Autodesk Fusion 360 part; units mm, degrees
(part 2 of 3)
sketch "slot_guide profile (3)" plane through (0, 0, -263) normal (0, 0, 1) x (1, 0, 0) in component "cassette_2 | Top cassette | DEPTH PROVISIONAL"
  line L0 (173, 552) -> (175, 552)
  line L1 (175, 552) -> (175, 554)
  line L2 (175, 554) -> (173, 554)
  line L3 (173, 554) -> (173, 552)
  line L4 (201, 552) -> (203, 552)
  line L5 (203, 552) -> (203, 554)
  line L6 (203, 554) -> (201, 554)
  line L7 (201, 554) -> (201, 552)
  line L8 (173, 541.5) -> (175, 541.5)
  line L9 (175, 541.5) -> (175, 543.5)
  line L10 (175, 543.5) -> (173, 543.5)
  line L11 (173, 543.5) -> (173, 541.5)
  line L12 (201, 541.5) -> (203, 541.5)
  line L13 (203, 541.5) -> (203, 543.5)
  line L14 (203, 543.5) -> (201, 543.5)
  line L15 (201, 543.5) -> (201, 541.5)
  line L16 (173, 531) -> (175, 531)
  line L17 (175, 531) -> (175, 533)
  line L18 (175, 533) -> (173, 533)
  line L19 (173, 533) -> (173, 531)
  line L20 (201, 531) -> (203, 531)
  line L21 (203, 531) -> (203, 533)
  line L22 (203, 533) -> (201, 533)
  line L23 (201, 533) -> (201, 531)
  line L24 (173, 520.5) -> (175, 520.5)
  line L25 (175, 520.5) -> (175, 522.5)
  line L26 (175, 522.5) -> (173, 522.5)
  line L27 (173, 522.5) -> (173, 520.5)
  line L28 (201, 520.5) -> (203, 520.5)
  line L29 (203, 520.5) -> (203, 522.5)
  line L30 (203, 522.5) -> (201, 522.5)
  line L31 (201, 522.5) -> (201, 520.5)
  line L32 (173, 510) -> (175, 510)
  line L33 (175, 510) -> (175, 512)
  line L34 (175, 512) -> (173, 512)
  line L35 (173, 512) -> (173, 510)
  line L36 (201, 510) -> (203, 510)
  line L37 (203, 510) -> (203, 512)
  line L38 (203, 512) -> (201, 512)
  line L39 (201, 512) -> (201, 510)
  line L40 (173, 499.5) -> (175, 499.5)
  line L41 (175, 499.5) -> (175, 501.5)
  line L42 (175, 501.5) -> (173, 501.5)
  line L43 (173, 501.5) -> (173, 499.5)
  line L44 (201, 499.5) -> (203, 499.5)
  line L45 (203, 499.5) -> (203, 501.5)
  line L46 (203, 501.5) -> (201, 501.5)
  line L47 (201, 501.5) -> (201, 499.5)
  line L48 (173, 489) -> (175, 489)
  line L49 (175, 489) -> (175, 491)
  line L50 (175, 491) -> (173, 491)
  line L51 (173, 491) -> (173, 489)
  line L52 (201, 489) -> (203, 489)
  line L53 (203, 489) -> (203, 491)
  line L54 (203, 491) -> (201, 491)
  line L55 (201, 491) -> (201, 489)
  line L56 (173, 478.5) -> (175, 478.5)
  line L57 (175, 478.5) -> (175, 480.5)
  line L58 (175, 480.5) -> (173, 480.5)
  line L59 (173, 480.5) -> (173, 478.5)
  line L60 (201, 478.5) -> (203, 478.5)
  line L61 (203, 478.5) -> (203, 480.5)
  line L62 (203, 480.5) -> (201, 480.5)
  line L63 (201, 480.5) -> (201, 478.5)
  line L64 (173, 468) -> (175, 468)
  line L65 (175, 468) -> (175, 470)
  line L66 (175, 470) -> (173, 470)
  line L67 (173, 470) -> (173, 468)
  line L68 (201, 468) -> (203, 468)
  line L69 (203, 468) -> (203, 470)
  line L70 (203, 470) -> (201, 470)
  line L71 (201, 470) -> (201, 468)
  line L72 (173, 457.5) -> (175, 457.5)
  line L73 (175, 457.5) -> (175, 459.5)
  line L74 (175, 459.5) -> (173, 459.5)
  line L75 (173, 459.5) -> (173, 457.5)
  line L76 (201, 457.5) -> (203, 457.5)
  line L77 (203, 457.5) -> (203, 459.5)
  line L78 (203, 459.5) -> (201, 459.5)
  line L79 (201, 459.5) -> (201, 457.5)
  line L80 (207, 552) -> (209, 552)
  line L81 (209, 552) -> (209, 554)
  line L82 (209, 554) -> (207, 554)
  line L83 (207, 554) -> (207, 552)
  line L84 (235, 552) -> (237, 552)
  line L85 (237, 552) -> (237, 554)
  line L86 (237, 554) -> (235, 554)
  line L87 (235, 554) -> (235, 552)
  line L88 (207, 541.5) -> (209, 541.5)
  line L89 (209, 541.5) -> (209, 543.5)
  line L90 (209, 543.5) -> (207, 543.5)
  line L91 (207, 543.5) -> (207, 541.5)
  line L92 (235, 541.5) -> (237, 541.5)
  line L93 (237, 541.5) -> (237, 543.5)
  line L94 (237, 543.5) -> (235, 543.5)
  line L95 (235, 543.5) -> (235, 541.5)
  line L96 (207, 531) -> (209, 531)
  line L97 (209, 531) -> (209, 533)
  line L98 (209, 533) -> (207, 533)
  line L99 (207, 533) -> (207, 531)
  line L100 (235, 531) -> (237, 531)
  line L101 (237, 531) -> (237, 533)
  line L102 (237, 533) -> (235, 533)
  line L103 (235, 533) -> (235, 531)
  line L104 (207, 520.5) -> (209, 520.5)
  line L105 (209, 520.5) -> (209, 522.5)
  line L106 (209, 522.5) -> (207, 522.5)
  line L107 (207, 522.5) -> (207, 520.5)
  line L108 (235, 520.5) -> (237, 520.5)
  line L109 (237, 520.5) -> (237, 522.5)
  line L110 (237, 522.5) -> (235, 522.5)
  line L111 (235, 522.5) -> (235, 520.5)
  line L112 (207, 510) -> (209, 510)
  line L113 (209, 510) -> (209, 512)
  line L114 (209, 512) -> (207, 512)
  line L115 (207, 512) -> (207, 510)
  line L116 (235, 510) -> (237, 510)
  line L117 (237, 510) -> (237, 512)
  line L118 (237, 512) -> (235, 512)
  line L119 (235, 512) -> (235, 510)
  line L120 (207, 499.5) -> (209, 499.5)
  line L121 (209, 499.5) -> (209, 501.5)
  line L122 (209, 501.5) -> (207, 501.5)
  line L123 (207, 501.5) -> (207, 499.5)
  line L124 (235, 499.5) -> (237, 499.5)
  line L125 (237, 499.5) -> (237, 501.5)
  line L126 (237, 501.5) -> (235, 501.5)
  line L127 (235, 501.5) -> (235, 499.5)
  line L128 (207, 489) -> (209, 489)
  line L129 (209, 489) -> (209, 491)
  line L130 (209, 491) -> (207, 491)
  line L131 (207, 491) -> (207, 489)
  line L132 (235, 489) -> (237, 489)
  line L133 (237, 489) -> (237, 491)
  line L134 (237, 491) -> (235, 491)
  line L135 (235, 491) -> (235, 489)
  line L136 (207, 478.5) -> (209, 478.5)
  line L137 (209, 478.5) -> (209, 480.5)
  line L138 (209, 480.5) -> (207, 480.5)
  line L139 (207, 480.5) -> (207, 478.5)
  line L140 (235, 478.5) -> (237, 478.5)
  line L141 (237, 478.5) -> (237, 480.5)
  line L142 (237, 480.5) -> (235, 480.5)
  line L143 (235, 480.5) -> (235, 478.5)
  line L144 (207, 468) -> (209, 468)
  line L145 (209, 468) -> (209, 470)
  line L146 (209, 470) -> (207, 470)
  line L147 (207, 470) -> (207, 468)
  line L148 (235, 468) -> (237, 468)
  line L149 (237, 468) -> (237, 470)
  line L150 (237, 470) -> (235, 470)
  line L151 (235, 470) -> (235, 468)
  line L152 (207, 457.5) -> (209, 457.5)
  line L153 (209, 457.5) -> (209, 459.5)
  line L154 (209, 459.5) -> (207, 459.5)
  line L155 (207, 459.5) -> (207, 457.5)
  line L156 (235, 457.5) -> (237, 457.5)
  line L157 (237, 457.5) -> (237, 459.5)
  line L158 (237, 459.5) -> (235, 459.5)
  line L159 (235, 459.5) -> (235, 457.5)
extrude "slot_guide solid extrusion''" add sketch "slot_guide profile (3)" along normal blind 83 separate body makes body 178 at (207, 458.8333, -207.6667) makes body 179 at (207, 469.3333, -207.6667) makes body 180 at (207, 479.8333, -207.6667) makes body 181 at (207, 490.3333, -207.6667) makes body 182 at (207, 500.8333, -207.6667) makes body 183 at (207, 511.3333, -207.6667) makes body 184 at (207, 521.8333, -207.6667) makes body 185 at (207, 532.3333, -207.6667) makes body 186 at (207, 542.8333, -207.6667) makes body 187 at (207, 553.3333, -207.6667) makes body 188 at (201, 458.8333, -207.6667) makes body 189 at (201, 469.3333, -207.6667) makes body 190 at (201, 479.8333, -207.6667) makes body 191 at (201, 490.3333, -207.6667) makes body 192 at (201, 500.8333, -207.6667) makes body 193 at (201, 511.3333, -207.6667) makes body 194 at (201, 521.8333, -207.6667) makes body 195 at (201, 532.3333, -207.6667) makes body 196 at (201, 542.8333, -207.6667) makes body 197 at (201, 553.3333, -207.6667) makes body 198 at (173, 542.8333, -207.6667) makes body 199 at (173, 532.3333, -207.6667) makes body 200 at (173, 521.8333, -207.6667) makes body 201 at (173, 511.3333, -207.6667) makes body 202 at (173, 500.8333, -207.6667) makes body 203 at (173, 490.3333, -207.6667) makes body 204 at (173, 479.8333, -207.6667) makes body 205 at (173, 469.3333, -207.6667) makes body 206 at (173, 458.8333, -207.6667) makes body 207 at (173, 553.3333, -207.6667) makes body 208 at (235, 553.3333, -207.6667) makes body 209 at (235, 542.8333, -207.6667) makes body 210 at (235, 532.3333, -207.6667) makes body 211 at (235, 521.8333, -207.6667) makes body 212 at (235, 511.3333, -207.6667) makes body 213 at (235, 500.8333, -207.6667) makes body 214 at (235, 490.3333, -207.6667) makes body 215 at (235, 479.8333, -207.6667) makes body 216 at (235, 469.3333, -207.6667) makes body 217 at (235, 458.8333, -207.6667) in component "cassette_2 | Top cassette | DEPTH PROVISIONAL"
ref_plane "WorkPlane1" through (0, 0, -62.5) normal (0, 0, 1) x (1, 0, 0) in component "imaging_stage | Imaging stage (schematic)"
sketch "stage_base profile" plane through (0, 0, -62.5) normal (0, 0, 1) x (1, 0, 0) in component "imaging_stage | Imaging stage (schematic)"
  line L0 (-145, 251) -> (15, 251)
  line L1 (15, 251) -> (15, 269)
  line L2 (15, 269) -> (-145, 269)
  line L3 (-145, 269) -> (-145, 251)
extrude "stage_base solid extrusion" add sketch "stage_base profile" along normal blind 125 separate body makes body 218 in component "imaging_stage | Imaging stage (schematic)"
ref_plane "WorkPlane2" through (0, 0, -47.5) normal (0, 0, 1) x (1, 0, 0) in component "imaging_stage | Imaging stage (schematic)"
sketch "stage_plate profile" plane through (0, 0, -47.5) normal (0, 0, 1) x (1, 0, 0) in component "imaging_stage | Imaging stage (schematic)"
  line L0 (-121.5, 273) -> (-8.5, 273)
  line L1 (-8.5, 273) -> (-8.5, 283)
  line L2 (-8.5, 283) -> (-121.5, 283)
  line L3 (-121.5, 283) -> (-121.5, 273)
extrude "stage_plate solid extrusion" add sketch "stage_plate profile" along normal blind 95 separate body makes body 219 in component "imaging_stage | Imaging stage (schematic)"
ref_plane "WorkPlane3" through (0, 0, -41.5) normal (0, 0, 1) x (1, 0, 0) in component "imaging_stage | Imaging stage (schematic)"
sketch "glass_seat profile" plane through (0, 0, -41.5) normal (0, 0, 1) x (1, 0, 0) in component "imaging_stage | Imaging stage (schematic)"
  line L0 (-81.5, 283) -> (-48.5, 283)
  line L1 (-48.5, 283) -> (-48.5, 287)
  line L2 (-48.5, 287) -> (-81.5, 287)
  line L3 (-81.5, 287) -> (-81.5, 283)
extrude "glass_seat solid extrusion" add sketch "glass_seat profile" along normal blind 83 separate body makes body 220 in component "imaging_stage | Imaging stage (schematic)"
ref_plane "WorkPlane1" through (0, 0, -17) normal (0, 0, 1) x (1, 0, 0) in component "optics | Objective and condenser (schematic)"
sketch "objective_20x_NA075 profile" plane through (0, 0, -17) normal (0, 0, 1) x (1, 0, 0) in component "optics | Objective and condenser (schematic)"
  line L0 (-82, 186) -> (-48, 186)
  line L1 (-48, 186) -> (-48, 234)
  line L2 (-48, 234) -> (-82, 234)
  line L3 (-82, 234) -> (-82, 186)
extrude "objective_20x_NA075 solid extrusion" add sketch "objective_20x_NA075 profile" along normal blind 34 separate body makes body 221 in component "optics | Objective and condenser (schematic)"
ref_plane "WorkPlane2" through (0, 0, -24) normal (0, 0, 1) x (1, 0, 0) in component "optics | Objective and condenser (schematic)"
sketch "interchangeable_condenser profile" plane through (0, 0, -24) normal (0, 0, 1) x (1, 0, 0) in component "optics | Objective and condenser (schematic)"
  line L0 (-89, 332) -> (-41, 332)
  line L1 (-41, 332) -> (-41, 358)
  line L2 (-41, 358) -> (-89, 358)
  line L3 (-89, 358) -> (-89, 332)
extrude "interchangeable_condenser solid extrusion" add sketch "interchangeable_condenser profile" along normal blind 48 separate body makes body 222 in component "optics | Objective and condenser (schematic)"
ref_plane "WorkPlane1" through (0, 0, 157) normal (0, 0, 1) x (1, 0, 0) in component "calibration_storage | Calibration-slide compartment"
sketch "Four calibration storage slides - estimated placement" plane through (0, 0, 157) normal (0, 0, 1) x (1, 0, 0) in component "calibration_storage | Calibration-slide compartment"
  line L0 (-251, 194.5) -> (-225, 194.5)
  line L1 (-225, 194.5) -> (-225, 195.5)
  line L2 (-225, 195.5) -> (-251, 195.5)
  line L3 (-251, 195.5) -> (-251, 194.5)
  line L4 (-251, 209.5) -> (-225, 209.5)
  line L5 (-225, 209.5) -> (-225, 210.5)
  line L6 (-225, 210.5) -> (-251, 210.5)
  line L7 (-251, 210.5) -> (-251, 209.5)
  line L8 (-251, 224.5) -> (-225, 224.5)
  line L9 (-225, 224.5) -> (-225, 225.5)
  line L10 (-225, 225.5) -> (-251, 225.5)
  line L11 (-251, 225.5) -> (-251, 224.5)
  line L12 (-251, 239.5) -> (-225, 239.5)
  line L13 (-225, 239.5) -> (-225, 240.5)
  line L14 (-225, 240.5) -> (-251, 240.5)
  line L15 (-251, 240.5) -> (-251, 239.5)
extrude "Calibration slides (schematic)" add sketch "Four calibration storage slides - estimated placement" along normal blind 76 separate body makes body 223 at (-233.6667, 225.5, 182.3333) makes body 224 at (-233.6667, 210.5, 182.3333) makes body 225 at (-233.6667, 195.5, 182.3333) makes body 226 at (-233.6667, 240.5, 182.3333) in component "calibration_storage | Calibration-slide compartment"
ref_plane "WorkPlane1" through (0, 0, -325) normal (0, 0, 1) x (1, 0, 0) in component "base | Base and nominal envelope | revision 0.3"
sketch "base_plate profile" plane through (0, 0, -325) normal (0, 0, 1) x (1, 0, 0) in component "base | Base and nominal envelope | revision 0.3"
  line L0 (-325, 14) -> (325, 14)
  line L1 (325, 14) -> (325, 42)
  line L2 (325, 42) -> (-325, 42)
  line L3 (-325, 42) -> (-325, 14)
extrude "base_plate native extrusion" add sketch "base_plate profile" along normal blind 650 separate body makes body 227 in component "base | Base and nominal envelope | revision 0.3"
ref_plane "WorkPlane2" through (0, 0, -325) normal (0, 0, 1) x (1, 0, 0) in component "base | Base and nominal envelope | revision 0.3"
sketch "lower_body_band profile" plane through (0, 0, -325) normal (0, 0, 1) x (1, 0, 0) in component "base | Base and nominal envelope | revision 0.3"
  line L0 (-325, 42) -> (325, 42)
  line L1 (325, 42) -> (325, 98)
  line L2 (325, 98) -> (-325, 98)
  line L3 (-325, 98) -> (-325, 42)
extrude "lower_body_band native extrusion" add sketch "lower_body_band profile" along normal blind 650 separate body makes body 228 in component "base | Base and nominal envelope | revision 0.3"
ref_plane "WorkPlane3" through (0, 0, -282.5) normal (0, 0, 1) x (1, 0, 0) in component "base | Base and nominal envelope | revision 0.3"
sketch "foot profile" plane through (0, 0, -282.5) normal (0, 0, 1) x (1, 0, 0) in component "base | Base and nominal envelope | revision 0.3"
  line L0 (-302.5, 0) -> (-267.5, 0)
  line L1 (-267.5, 0) -> (-267.5, 14)
  line L2 (-267.5, 14) -> (-302.5, 14)
  line L3 (-302.5, 14) -> (-302.5, 0)
  line L4 (267.5, 0) -> (302.5, 0)
  line L5 (302.5, 0) -> (302.5, 14)
  line L6 (302.5, 14) -> (267.5, 14)
  line L7 (267.5, 14) -> (267.5, 0)
extrude "foot native extrusion" add sketch "foot profile" along normal blind 35 separate body makes body 229 at (-279.1667, 14, -270.8333) makes body 230 at (290.8333, 14, -270.8333) in component "base | Base and nominal envelope | revision 0.3"
ref_plane "WorkPlane4" through (0, 0, 247.5) normal (0, 0, 1) x (1, 0, 0) in component "base | Base and nominal envelope | revision 0.3"
sketch "foot profile (1)" plane through (0, 0, 247.5) normal (0, 0, 1) x (1, 0, 0) in component "base | Base and nominal envelope | revision 0.3"
  line L0 (-302.5, 0) -> (-267.5, 0)
  line L1 (-267.5, 0) -> (-267.5, 14)
  line L2 (-267.5, 14) -> (-302.5, 14)
  line L3 (-302.5, 14) -> (-302.5, 0)
  line L4 (267.5, 0) -> (302.5, 0)
  line L5 (302.5, 0) -> (302.5, 14)
  line L6 (302.5, 14) -> (267.5, 14)
  line L7 (267.5, 14) -> (267.5, 0)
extrude "foot native extrusion (1)" add sketch "foot profile (1)" along normal blind 35 separate body makes body 231 at (-279.1667, 14, 259.1667) makes body 232 at (290.8333, 14, 259.1667) in component "base | Base and nominal envelope | revision 0.3"
ref_plane "WorkPlane1" through (0, 0, -311) normal (0, 0, 1) x (1, 0, 0) in component "enclosure | Enclosure - revised silhouette | revision 0.3"
sketch "rounded_casing measured-outline reference" plane through (0, 0, -311) normal (0, 0, 1) x (1, 0, 0) in component "enclosure | Enclosure - revised silhouette | revision 0.3"
  line L0 (-325, 70) -> (325, 70)
  line L1 (325, 70) -> (325, 610)
  arc A0 (325, 610) -> (235, 700) centre (235, 610) ccw
  line L2 (235, 700) -> (-325, 700)
  line L3 (-325, 700) -> (-325, 70)
  line L4 (-311, 84) -> (-311, 686)
  line L5 (-311, 686) -> (235, 686)
  arc A1 (311, 610) -> (235, 686) centre (235, 610) ccw
  line L6 (311, 610) -> (311, 84)
  line L7 (311, 84) -> (-311, 84)
extrude "rounded_casing native extrusion" add sketch "rounded_casing measured-outline reference" along normal blind 636 separate body makes body 233 in component "enclosure | Enclosure - revised silhouette | revision 0.3"
ref_plane "WorkPlane2" through (0, 0, -325) normal (0, 0, 1) x (1, 0, 0) in component "enclosure | Enclosure - revised silhouette | revision 0.3"
sketch "rear_panel measured-outline reference" plane through (0, 0, -325) normal (0, 0, 1) x (1, 0, 0) in component "enclosure | Enclosure - revised silhouette | revision 0.3"
  line L0 (-325, 70) -> (325, 70)
  line L1 (325, 70) -> (325, 610)
  arc A0 (325, 610) -> (235, 700) centre (235, 610) ccw
  line L2 (235, 700) -> (-325, 700)
  line L3 (-325, 700) -> (-325, 70)
extrude "rear_panel native extrusion" add sketch "rear_panel measured-outline reference" along normal blind 14 separate body makes body 234 in component "enclosure | Enclosure - revised silhouette | revision 0.3"
ref_plane "WorkPlane3" through (0, 0, 325) normal (0, 0, 1) x (1, 0, 0) in component "enclosure | Enclosure - revised silhouette | revision 0.3"
sketch "front_perimeter measured-outline reference" plane through (0, 0, 325) normal (0, 0, 1) x (1, 0, 0) in component "enclosure | Enclosure - revised silhouette | revision 0.3"
  line L0 (-325, 70) -> (325, 70)
  line L1 (325, 70) -> (325, 610)
  arc A0 (325, 610) -> (235, 700) centre (235, 610) ccw
  line L2 (235, 700) -> (-325, 700)
  line L3 (-325, 700) -> (-325, 70)
  line L4 (-311, 84) -> (-311, 686)
  line L5 (-311, 686) -> (235, 686)
  arc A1 (311, 610) -> (235, 686) centre (235, 610) ccw
  line L6 (311, 610) -> (311, 84)
  line L7 (311, 84) -> (-311, 84)
extrude "front_perimeter native extrusion" add sketch "front_perimeter measured-outline reference" along normal blind 7 separate body makes body 235 in component "enclosure | Enclosure - revised silhouette | revision 0.3"
ref_plane "WorkPlane4" through (0, 0, 346) normal (0, 0, 1) x (1, 0, 0) in component "enclosure | Enclosure - revised silhouette | revision 0.3"
sketch "fixed_front_notched measured-outline reference" plane through (0, 0, 346) normal (0, 0, 1) x (1, 0, 0) in component "enclosure | Enclosure - revised silhouette | revision 0.3"
  line L0 (-311, 119) -> (62, 119)
  line L1 (62, 119) -> (62, 333)
  line L2 (62, 333) -> (30, 365)
  line L3 (30, 365) -> (30, 475)
  line L4 (30, 475) -> (62, 507)
  line L5 (62, 507) -> (62, 686)
  line L6 (62, 686) -> (-311, 686)
  line L7 (-311, 686) -> (-311, 119)
extrude "fixed_front_notched native extrusion" add sketch "fixed_front_notched measured-outline reference" along normal blind 8 separate body makes body 236 in component "enclosure | Enclosure - revised silhouette | revision 0.3"
ref_plane "WorkPlane5" through (0, 0, 325) normal (0, 0, 1) x (1, 0, 0) in component "enclosure | Enclosure - revised silhouette | revision 0.3"
sketch "front_sill profile" plane through (0, 0, 325) normal (0, 0, 1) x (1, 0, 0) in component "enclosure | Enclosure - revised silhouette | revision 0.3"
  line L0 (-325, 98) -> (325, 98)
  line L1 (325, 98) -> (325, 119)
  line L2 (325, 119) -> (-325, 119)
  line L3 (-325, 119) -> (-325, 98)
extrude "front_sill native extrusion" add sketch "front_sill profile" along normal blind 22 separate body makes body 237 in component "enclosure | Enclosure - revised silhouette | revision 0.3"
ref_plane "WorkPlane6" through (0, 0, 308) normal (0, 0, 1) x (1, 0, 0) in component "enclosure | Enclosure - revised silhouette | revision 0.3"
sketch "left_service_hinge profile" plane through (0, 0, 308) normal (0, 0, 1) x (1, 0, 0) in component "enclosure | Enclosure - revised silhouette | revision 0.3"
  line L0 (-343, 131) -> (-321, 131)
  line L1 (-321, 131) -> (-321, 159)
  line L2 (-321, 159) -> (-343, 159)
  line L3 (-343, 159) -> (-343, 131)
  line L4 (-343, 606) -> (-321, 606)
  line L5 (-321, 606) -> (-321, 634)
  line L6 (-321, 634) -> (-343, 634)
  line L7 (-343, 634) -> (-343, 606)
extrude "left_service_hinge native extrusion" add sketch "left_service_hinge profile" along normal blind 12 separate body makes body 238 at (-335.6667, 140.3333, 308) makes body 239 at (-335.6667, 615.3333, 308) in component "enclosure | Enclosure - revised silhouette | revision 0.3"
ref_plane "WorkPlane7" through (0, 0, 227.5) normal (0, 0, 1) x (1, 0, 0) in component "enclosure | Enclosure - revised silhouette | revision 0.3"
sketch "right_service_latch profile" plane through (0, 0, 227.5) normal (0, 0, 1) x (1, 0, 0) in component "enclosure | Enclosure - revised silhouette | revision 0.3"
  line L0 (325, 137.5) -> (342, 137.5)
  line L1 (342, 137.5) -> (342, 152.5)
  line L2 (342, 152.5) -> (325, 152.5)
  line L3 (325, 152.5) -> (325, 137.5)
  line L4 (325, 612.5) -> (342, 612.5)
  line L5 (342, 612.5) -> (342, 627.5)
  line L6 (342, 627.5) -> (325, 627.5)
  line L7 (325, 627.5) -> (325, 612.5)
extrude "right_service_latch native extrusion" add sketch "right_service_latch profile" along normal blind 25 separate body makes body 240 at (336.3333, 152.5, 235.8333) makes body 241 at (336.3333, 627.5, 235.8333) in component "enclosure | Enclosure - revised silhouette | revision 0.3"
ref_plane "WorkPlane8" through (0, 0, -296) normal (0, 0, 1) x (1, 0, 0) in component "enclosure | Enclosure - revised silhouette | revision 0.3"
sketch "right_service_panel profile" plane through (0, 0, -296) normal (0, 0, 1) x (1, 0, 0) in component "enclosure | Enclosure - revised silhouette | revision 0.3"
  line L0 (324, 129) -> (326, 129)
  line L1 (326, 129) -> (326, 537)
  line L2 (326, 537) -> (324, 537)
  line L3 (324, 537) -> (324, 129)
extrude "right_service_panel native extrusion" add sketch "right_service_panel profile" along normal blind 410 separate body makes body 242 in component "enclosure | Enclosure - revised silhouette | revision 0.3"
ref_plane "WorkPlane9" through (0, 0, -19) normal (0, 0, 1) x (1, 0, 0) in component "enclosure | Enclosure - revised silhouette | revision 0.3"
sketch "right_service_handle profile" plane through (0, 0, -19) normal (0, 0, 1) x (1, 0, 0) in component "enclosure | Enclosure - revised silhouette | revision 0.3"
  line L0 (326, 305.5) -> (338, 305.5)
  line L1 (338, 305.5) -> (338, 390.5)
  line L2 (338, 390.5) -> (326, 390.5)
  line L3 (326, 390.5) -> (326, 305.5)
extrude "right_service_handle native extrusion" add sketch "right_service_handle profile" along normal blind 24 separate body makes body 243 in component "enclosure | Enclosure - revised silhouette | revision 0.3"
ref_plane "WorkPlane10" through (0, 0, -282.5) normal (0, 0, 1) x (1, 0, 0) in component "enclosure | Enclosure - revised silhouette | revision 0.3"
sketch "side_vent profile" plane through (0, 0, -282.5) normal (0, 0, 1) x (1, 0, 0) in component "enclosure | Enclosure - revised silhouette | revision 0.3"
  line L0 (324.5, 106.5) -> (326.5, 106.5)
  line L1 (326.5, 106.5) -> (326.5, 109.5)
  line L2 (326.5, 109.5) -> (324.5, 109.5)
  line L3 (324.5, 109.5) -> (324.5, 106.5)
  line L4 (324.5, 117.5) -> (326.5, 117.5)
  line L5 (326.5, 117.5) -> (326.5, 120.5)
  line L6 (326.5, 120.5) -> (324.5, 120.5)
  line L7 (324.5, 120.5) -> (324.5, 117.5)
  line L8 (324.5, 128.5) -> (326.5, 128.5)
  line L9 (326.5, 128.5) -> (326.5, 131.5)
  line L10 (326.5, 131.5) -> (324.5, 131.5)
  line L11 (324.5, 131.5) -> (324.5, 128.5)
  line L12 (324.5, 139.5) -> (326.5, 139.5)
  line L13 (326.5, 139.5) -> (326.5, 142.5)
  line L14 (326.5, 142.5) -> (324.5, 142.5)
  line L15 (324.5, 142.5) -> (324.5, 139.5)
  line L16 (324.5, 150.5) -> (326.5, 150.5)
  line L17 (326.5, 150.5) -> (326.5, 153.5)
  line L18 (326.5, 153.5) -> (324.5, 153.5)
  line L19 (324.5, 153.5) -> (324.5, 150.5)
extrude "side_vent native extrusion" add sketch "side_vent profile" along normal blind 5 separate body makes body 244 at (324.5, 141.5, -280.8333) makes body 245 at (324.5, 130.5, -280.8333) makes body 246 at (324.5, 119.5, -280.8333) makes body 247 at (324.5, 108.5, -280.8333) makes body 248 at (324.5, 152.5, -280.8333) in component "enclosure | Enclosure - revised silhouette | revision 0.3"
ref_plane "WorkPlane11" through (0, 0, -254.5) normal (0, 0, 1) x (1, 0, 0) in component "enclosure | Enclosure - revised silhouette | revision 0.3"
sketch "side_vent profile (1)" plane through (0, 0, -254.5) normal (0, 0, 1) x (1, 0, 0) in component "enclosure | Enclosure - revised silhouette | revision 0.3"
  line L0 (324.5, 106.5) -> (326.5, 106.5)
  line L1 (326.5, 106.5) -> (326.5, 109.5)
  line L2 (326.5, 109.5) -> (324.5, 109.5)
  line L3 (324.5, 109.5) -> (324.5, 106.5)
  line L4 (324.5, 117.5) -> (326.5, 117.5)
  line L5 (326.5, 117.5) -> (326.5, 120.5)
  line L6 (326.5, 120.5) -> (324.5, 120.5)
  line L7 (324.5, 120.5) -> (324.5, 117.5)
  line L8 (324.5, 128.5) -> (326.5, 128.5)
  line L9 (326.5, 128.5) -> (326.5, 131.5)
  line L10 (326.5, 131.5) -> (324.5, 131.5)
  line L11 (324.5, 131.5) -> (324.5, 128.5)
  line L12 (324.5, 139.5) -> (326.5, 139.5)
  line L13 (326.5, 139.5) -> (326.5, 142.5)
  line L14 (326.5, 142.5) -> (324.5, 142.5)
  line L15 (324.5, 142.5) -> (324.5, 139.5)
  line L16 (324.5, 150.5) -> (326.5, 150.5)
  line L17 (326.5, 150.5) -> (326.5, 153.5)
  line L18 (326.5, 153.5) -> (324.5, 153.5)
  line L19 (324.5, 153.5) -> (324.5, 150.5)
extrude "side_vent native extrusion (1)" add sketch "side_vent profile (1)" along normal blind 5 separate body makes body 249 at (324.5, 141.5, -252.8333) makes body 250 at (324.5, 130.5, -252.8333) makes body 251 at (324.5, 119.5, -252.8333) makes body 252 at (324.5, 108.5, -252.8333) makes body 253 at (324.5, 152.5, -252.8333) in component "enclosure | Enclosure - revised silhouette | revision 0.3"
ref_plane "WorkPlane12" through (0, 0, -226.5) normal (0, 0, 1) x (1, 0, 0) in component "enclosure | Enclosure - revised silhouette | revision 0.3"
sketch "side_vent profile (2)" plane through (0, 0, -226.5) normal (0, 0, 1) x (1, 0, 0) in component "enclosure | Enclosure - revised silhouette | revision 0.3"
  line L0 (324.5, 106.5) -> (326.5, 106.5)
  line L1 (326.5, 106.5) -> (326.5, 109.5)
  line L2 (326.5, 109.5) -> (324.5, 109.5)
  line L3 (324.5, 109.5) -> (324.5, 106.5)
  line L4 (324.5, 117.5) -> (326.5, 117.5)
  line L5 (326.5, 117.5) -> (326.5, 120.5)
  line L6 (326.5, 120.5) -> (324.5, 120.5)
  line L7 (324.5, 120.5) -> (324.5, 117.5)
  line L8 (324.5, 128.5) -> (326.5, 128.5)
  line L9 (326.5, 128.5) -> (326.5, 131.5)
  line L10 (326.5, 131.5) -> (324.5, 131.5)
  line L11 (324.5, 131.5) -> (324.5, 128.5)
  line L12 (324.5, 139.5) -> (326.5, 139.5)
  line L13 (326.5, 139.5) -> (326.5, 142.5)
  line L14 (326.5, 142.5) -> (324.5, 142.5)
  line L15 (324.5, 142.5) -> (324.5, 139.5)
  line L16 (324.5, 150.5) -> (326.5, 150.5)
  line L17 (326.5, 150.5) -> (326.5, 153.5)
  line L18 (326.5, 153.5) -> (324.5, 153.5)
  line L19 (324.5, 153.5) -> (324.5, 150.5)
extrude "side_vent native extrusion (2)" add sketch "side_vent profile (2)" along normal blind 5 separate body makes body 254 at (324.5, 141.5, -224.8333) makes body 255 at (324.5, 130.5, -224.8333) makes body 256 at (324.5, 119.5, -224.8333) makes body 257 at (324.5, 108.5, -224.8333) makes body 258 at (324.5, 152.5, -224.8333) in component "enclosure | Enclosure - revised silhouette | revision 0.3"
ref_plane "WorkPlane13" through (0, 0, -198.5) normal (0, 0, 1) x (1, 0, 0) in component "enclosure | Enclosure - revised silhouette | revision 0.3"
sketch "side_vent profile (3)" plane through (0, 0, -198.5) normal (0, 0, 1) x (1, 0, 0) in component "enclosure | Enclosure - revised silhouette | revision 0.3"
  line L0 (324.5, 106.5) -> (326.5, 106.5)
  line L1 (326.5, 106.5) -> (326.5, 109.5)
  line L2 (326.5, 109.5) -> (324.5, 109.5)
  line L3 (324.5, 109.5) -> (324.5, 106.5)
  line L4 (324.5, 117.5) -> (326.5, 117.5)
  line L5 (326.5, 117.5) -> (326.5, 120.5)
  line L6 (326.5, 120.5) -> (324.5, 120.5)
  line L7 (324.5, 120.5) -> (324.5, 117.5)
  line L8 (324.5, 128.5) -> (326.5, 128.5)
  line L9 (326.5, 128.5) -> (326.5, 131.5)
  line L10 (326.5, 131.5) -> (324.5, 131.5)
  line L11 (324.5, 131.5) -> (324.5, 128.5)
  line L12 (324.5, 139.5) -> (326.5, 139.5)
  line L13 (326.5, 139.5) -> (326.5, 142.5)
  line L14 (326.5, 142.5) -> (324.5, 142.5)
  line L15 (324.5, 142.5) -> (324.5, 139.5)
  line L16 (324.5, 150.5) -> (326.5, 150.5)
  line L17 (326.5, 150.5) -> (326.5, 153.5)
  line L18 (326.5, 153.5) -> (324.5, 153.5)
  line L19 (324.5, 153.5) -> (324.5, 150.5)
extrude "side_vent native extrusion (3)" add sketch "side_vent profile (3)" along normal blind 5 separate body makes body 259 at (324.5, 141.5, -196.8333) makes body 260 at (324.5, 130.5, -196.8333) makes body 261 at (324.5, 119.5, -196.8333) makes body 262 at (324.5, 108.5, -196.8333) makes body 263 at (324.5, 152.5, -196.8333) in component "enclosure | Enclosure - revised silhouette | revision 0.3"
ref_plane "WorkPlane14" through (0, 0, -170.5) normal (0, 0, 1) x (1, 0, 0) in component "enclosure | Enclosure - revised silhouette | revision 0.3"
sketch "side_vent profile (4)" plane through (0, 0, -170.5) normal (0, 0, 1) x (1, 0, 0) in component "enclosure | Enclosure - revised silhouette | revision 0.3"
  line L0 (324.5, 106.5) -> (326.5, 106.5)
  line L1 (326.5, 106.5) -> (326.5, 109.5)
  line L2 (326.5, 109.5) -> (324.5, 109.5)
  line L3 (324.5, 109.5) -> (324.5, 106.5)
  line L4 (324.5, 117.5) -> (326.5, 117.5)
  line L5 (326.5, 117.5) -> (326.5, 120.5)
  line L6 (326.5, 120.5) -> (324.5, 120.5)
  line L7 (324.5, 120.5) -> (324.5, 117.5)
  line L8 (324.5, 128.5) -> (326.5, 128.5)
  line L9 (326.5, 128.5) -> (326.5, 131.5)
  line L10 (326.5, 131.5) -> (324.5, 131.5)
  line L11 (324.5, 131.5) -> (324.5, 128.5)
  line L12 (324.5, 139.5) -> (326.5, 139.5)
  line L13 (326.5, 139.5) -> (326.5, 142.5)
  line L14 (326.5, 142.5) -> (324.5, 142.5)
  line L15 (324.5, 142.5) -> (324.5, 139.5)
  line L16 (324.5, 150.5) -> (326.5, 150.5)
  line L17 (326.5, 150.5) -> (326.5, 153.5)
  line L18 (326.5, 153.5) -> (324.5, 153.5)
  line L19 (324.5, 153.5) -> (324.5, 150.5)
extrude "side_vent native extrusion (4)" add sketch "side_vent profile (4)" along normal blind 5 separate body makes body 264 at (324.5, 141.5, -168.8333) makes body 265 at (324.5, 130.5, -168.8333) makes body 266 at (324.5, 119.5, -168.8333) makes body 267 at (324.5, 108.5, -168.8333) makes body 268 at (324.5, 152.5, -168.8333) in component "enclosure | Enclosure - revised silhouette | revision 0.3"
ref_plane "WorkPlane15" through (0, 0, -142.5) normal (0, 0, 1) x (1, 0, 0) in component "enclosure | Enclosure - revised silhouette | revision 0.3"
sketch "side_vent profile (5)" plane through (0, 0, -142.5) normal (0, 0, 1) x (1, 0, 0) in component "enclosure | Enclosure - revised silhouette | revision 0.3"
  line L0 (324.5, 106.5) -> (326.5, 106.5)
  line L1 (326.5, 106.5) -> (326.5, 109.5)
  line L2 (326.5, 109.5) -> (324.5, 109.5)
  line L3 (324.5, 109.5) -> (324.5, 106.5)
  line L4 (324.5, 117.5) -> (326.5, 117.5)
  line L5 (326.5, 117.5) -> (326.5, 120.5)
  line L6 (326.5, 120.5) -> (324.5, 120.5)
  line L7 (324.5, 120.5) -> (324.5, 117.5)
  line L8 (324.5, 128.5) -> (326.5, 128.5)
  line L9 (326.5, 128.5) -> (326.5, 131.5)
  line L10 (326.5, 131.5) -> (324.5, 131.5)
  line L11 (324.5, 131.5) -> (324.5, 128.5)
  line L12 (324.5, 139.5) -> (326.5, 139.5)
  line L13 (326.5, 139.5) -> (326.5, 142.5)
  line L14 (326.5, 142.5) -> (324.5, 142.5)
  line L15 (324.5, 142.5) -> (324.5, 139.5)
  line L16 (324.5, 150.5) -> (326.5, 150.5)
  line L17 (326.5, 150.5) -> (326.5, 153.5)
  line L18 (326.5, 153.5) -> (324.5, 153.5)
  line L19 (324.5, 153.5) -> (324.5, 150.5)
extrude "side_vent native extrusion (5)" add sketch "side_vent profile (5)" along normal blind 5 separate body makes body 269 at (324.5, 141.5, -140.8333) makes body 270 at (324.5, 130.5, -140.8333) makes body 271 at (324.5, 119.5, -140.8333) makes body 272 at (324.5, 108.5, -140.8333) makes body 273 at (324.5, 152.5, -140.8333) in component "enclosure | Enclosure - revised silhouette | revision 0.3"
ref_plane "WorkPlane16" through (0, 0, -114.5) normal (0, 0, 1) x (1, 0, 0) in component "enclosure | Enclosure - revised silhouette | revision 0.3"
sketch "side_vent profile (6)" plane through (0, 0, -114.5) normal (0, 0, 1) x (1, 0, 0) in component "enclosure | Enclosure - revised silhouette | revision 0.3"
  line L0 (324.5, 106.5) -> (326.5, 106.5)
  line L1 (326.5, 106.5) -> (326.5, 109.5)
  line L2 (326.5, 109.5) -> (324.5, 109.5)
  line L3 (324.5, 109.5) -> (324.5, 106.5)
  line L4 (324.5, 117.5) -> (326.5, 117.5)
  line L5 (326.5, 117.5) -> (326.5, 120.5)
  line L6 (326.5, 120.5) -> (324.5, 120.5)
  line L7 (324.5, 120.5) -> (324.5, 117.5)
  line L8 (324.5, 128.5) -> (326.5, 128.5)
  line L9 (326.5, 128.5) -> (326.5, 131.5)
  line L10 (326.5, 131.5) -> (324.5, 131.5)
  line L11 (324.5, 131.5) -> (324.5, 128.5)
  line L12 (324.5, 139.5) -> (326.5, 139.5)
  line L13 (326.5, 139.5) -> (326.5, 142.5)
  line L14 (326.5, 142.5) -> (324.5, 142.5)
  line L15 (324.5, 142.5) -> (324.5, 139.5)
  line L16 (324.5, 150.5) -> (326.5, 150.5)
  line L17 (326.5, 150.5) -> (326.5, 153.5)
  line L18 (326.5, 153.5) -> (324.5, 153.5)
  line L19 (324.5, 153.5) -> (324.5, 150.5)
extrude "side_vent native extrusion (6)" add sketch "side_vent profile (6)" along normal blind 5 separate body makes body 274 at (324.5, 141.5, -112.8333) makes body 275 at (324.5, 130.5, -112.8333) makes body 276 at (324.5, 119.5, -112.8333) makes body 277 at (324.5, 108.5, -112.8333) makes body 278 at (324.5, 152.5, -112.8333) in component "enclosure | Enclosure - revised silhouette | revision 0.3"
ref_plane "WorkPlane17" through (0, 0, -86.5) normal (0, 0, 1) x (1, 0, 0) in component "enclosure | Enclosure - revised silhouette | revision 0.3"
sketch "side_vent profile (7)" plane through (0, 0, -86.5) normal (0, 0, 1) x (1, 0, 0) in component "enclosure | Enclosure - revised silhouette | revision 0.3"
  line L0 (324.5, 106.5) -> (326.5, 106.5)
  line L1 (326.5, 106.5) -> (326.5, 109.5)
  line L2 (326.5, 109.5) -> (324.5, 109.5)
  line L3 (324.5, 109.5) -> (324.5, 106.5)
  line L4 (324.5, 117.5) -> (326.5, 117.5)
  line L5 (326.5, 117.5) -> (326.5, 120.5)
  line L6 (326.5, 120.5) -> (324.5, 120.5)
  line L7 (324.5, 120.5) -> (324.5, 117.5)
  line L8 (324.5, 128.5) -> (326.5, 128.5)
  line L9 (326.5, 128.5) -> (326.5, 131.5)
  line L10 (326.5, 131.5) -> (324.5, 131.5)
  line L11 (324.5, 131.5) -> (324.5, 128.5)
  line L12 (324.5, 139.5) -> (326.5, 139.5)
  line L13 (326.5, 139.5) -> (326.5, 142.5)
  line L14 (326.5, 142.5) -> (324.5, 142.5)
  line L15 (324.5, 142.5) -> (324.5, 139.5)
  line L16 (324.5, 150.5) -> (326.5, 150.5)
  line L17 (326.5, 150.5) -> (326.5, 153.5)
  line L18 (326.5, 153.5) -> (324.5, 153.5)
  line L19 (324.5, 153.5) -> (324.5, 150.5)
extrude "side_vent native extrusion (7)" add sketch "side_vent profile (7)" along normal blind 5 separate body makes body 279 at (324.5, 141.5, -84.8333) makes body 280 at (324.5, 130.5, -84.8333) makes body 281 at (324.5, 119.5, -84.8333) makes body 282 at (324.5, 108.5, -84.8333) makes body 283 at (324.5, 152.5, -84.8333) in component "enclosure | Enclosure - revised silhouette | revision 0.3"
ref_plane "WorkPlane18" through (0, 0, -58.5) normal (0, 0, 1) x (1, 0, 0) in component "enclosure | Enclosure - revised silhouette | revision 0.3"
sketch "side_vent profile (8)" plane through (0, 0, -58.5) normal (0, 0, 1) x (1, 0, 0) in component "enclosure | Enclosure - revised silhouette | revision 0.3"
  line L0 (324.5, 106.5) -> (326.5, 106.5)
  line L1 (326.5, 106.5) -> (326.5, 109.5)
  line L2 (326.5, 109.5) -> (324.5, 109.5)
  line L3 (324.5, 109.5) -> (324.5, 106.5)
  line L4 (324.5, 117.5) -> (326.5, 117.5)
  line L5 (326.5, 117.5) -> (326.5, 120.5)
  line L6 (326.5, 120.5) -> (324.5, 120.5)
  line L7 (324.5, 120.5) -> (324.5, 117.5)
  line L8 (324.5, 128.5) -> (326.5, 128.5)
  line L9 (326.5, 128.5) -> (326.5, 131.5)
  line L10 (326.5, 131.5) -> (324.5, 131.5)
  line L11 (324.5, 131.5) -> (324.5, 128.5)
  line L12 (324.5, 139.5) -> (326.5, 139.5)
  line L13 (326.5, 139.5) -> (326.5, 142.5)
  line L14 (326.5, 142.5) -> (324.5, 142.5)
  line L15 (324.5, 142.5) -> (324.5, 139.5)
  line L16 (324.5, 150.5) -> (326.5, 150.5)
  line L17 (326.5, 150.5) -> (326.5, 153.5)
  line L18 (326.5, 153.5) -> (324.5, 153.5)
  line L19 (324.5, 153.5) -> (324.5, 150.5)
extrude "side_vent native extrusion (8)" add sketch "side_vent profile (8)" along normal blind 5 separate body makes body 284 at (324.5, 141.5, -56.8333) makes body 285 at (324.5, 130.5, -56.8333) makes body 286 at (324.5, 119.5, -56.8333) makes body 287 at (324.5, 108.5, -56.8333) makes body 288 at (324.5, 152.5, -56.8333) in component "enclosure | Enclosure - revised silhouette | revision 0.3"
ref_plane "WorkPlane19" through (0, 0, -30.5) normal (0, 0, 1) x (1, 0, 0) in component "enclosure | Enclosure - revised silhouette | revision 0.3"
sketch "side_vent profile (9)" plane through (0, 0, -30.5) normal (0, 0, 1) x (1, 0, 0) in component "enclosure | Enclosure - revised silhouette | revision 0.3"
  line L0 (324.5, 106.5) -> (326.5, 106.5)
  line L1 (326.5, 106.5) -> (326.5, 109.5)
  line L2 (326.5, 109.5) -> (324.5, 109.5)
  line L3 (324.5, 109.5) -> (324.5, 106.5)
  line L4 (324.5, 117.5) -> (326.5, 117.5)
  line L5 (326.5, 117.5) -> (326.5, 120.5)
  line L6 (326.5, 120.5) -> (324.5, 120.5)
  line L7 (324.5, 120.5) -> (324.5, 117.5)
  line L8 (324.5, 128.5) -> (326.5, 128.5)
  line L9 (326.5, 128.5) -> (326.5, 131.5)
  line L10 (326.5, 131.5) -> (324.5, 131.5)
  line L11 (324.5, 131.5) -> (324.5, 128.5)
  line L12 (324.5, 139.5) -> (326.5, 139.5)
  line L13 (326.5, 139.5) -> (326.5, 142.5)
  line L14 (326.5, 142.5) -> (324.5, 142.5)
  line L15 (324.5, 142.5) -> (324.5, 139.5)
  line L16 (324.5, 150.5) -> (326.5, 150.5)
  line L17 (326.5, 150.5) -> (326.5, 153.5)
  line L18 (326.5, 153.5) -> (324.5, 153.5)
  line L19 (324.5, 153.5) -> (324.5, 150.5)
extrude "side_vent native extrusion (9)" add sketch "side_vent profile (9)" along normal blind 5 separate body makes body 289 at (324.5, 141.5, -28.8333) makes body 290 at (324.5, 130.5, -28.8333) makes body 291 at (324.5, 119.5, -28.8333) makes body 292 at (324.5, 108.5, -28.8333) makes body 293 at (324.5, 152.5, -28.8333) in component "enclosure | Enclosure - revised silhouette | revision 0.3"
ref_plane "WorkPlane20" through (0, 0, -2.5) normal (0, 0, 1) x (1, 0, 0) in component "enclosure | Enclosure - revised silhouette | revision 0.3"
sketch "side_vent profile (10)" plane through (0, 0, -2.5) normal (0, 0, 1) x (1, 0, 0) in component "enclosure | Enclosure - revised silhouette | revision 0.3"
  line L0 (324.5, 106.5) -> (326.5, 106.5)
  line L1 (326.5, 106.5) -> (326.5, 109.5)
  line L2 (326.5, 109.5) -> (324.5, 109.5)
  line L3 (324.5, 109.5) -> (324.5, 106.5)
  line L4 (324.5, 117.5) -> (326.5, 117.5)
  line L5 (326.5, 117.5) -> (326.5, 120.5)
  line L6 (326.5, 120.5) -> (324.5, 120.5)
  line L7 (324.5, 120.5) -> (324.5, 117.5)
  line L8 (324.5, 128.5) -> (326.5, 128.5)
  line L9 (326.5, 128.5) -> (326.5, 131.5)
  line L10 (326.5, 131.5) -> (324.5, 131.5)
  line L11 (324.5, 131.5) -> (324.5, 128.5)
  line L12 (324.5, 139.5) -> (326.5, 139.5)
  line L13 (326.5, 139.5) -> (326.5, 142.5)
  line L14 (326.5, 142.5) -> (324.5, 142.5)
  line L15 (324.5, 142.5) -> (324.5, 139.5)
  line L16 (324.5, 150.5) -> (326.5, 150.5)
  line L17 (326.5, 150.5) -> (326.5, 153.5)
  line L18 (326.5, 153.5) -> (324.5, 153.5)
  line L19 (324.5, 153.5) -> (324.5, 150.5)
extrude "side_vent native extrusion (10)" add sketch "side_vent profile (10)" along normal blind 5 separate body makes body 294 at (324.5, 141.5, -0.8333) makes body 295 at (324.5, 130.5, -0.8333) makes body 296 at (324.5, 119.5, -0.8333) makes body 297 at (324.5, 108.5, -0.8333) makes body 298 at (324.5, 152.5, -0.8333) in component "enclosure | Enclosure - revised silhouette | revision 0.3"
ref_plane "WorkPlane21" through (0, 0, 25.5) normal (0, 0, 1) x (1, 0, 0) in component "enclosure | Enclosure - revised silhouette | revision 0.3"
sketch "side_vent profile (11)" plane through (0, 0, 25.5) normal (0, 0, 1) x (1, 0, 0) in component "enclosure | Enclosure - revised silhouette | revision 0.3"
  line L0 (324.5, 106.5) -> (326.5, 106.5)
  line L1 (326.5, 106.5) -> (326.5, 109.5)
  line L2 (326.5, 109.5) -> (324.5, 109.5)
  line L3 (324.5, 109.5) -> (324.5, 106.5)
  line L4 (324.5, 117.5) -> (326.5, 117.5)
  line L5 (326.5, 117.5) -> (326.5, 120.5)
  line L6 (326.5, 120.5) -> (324.5, 120.5)
  line L7 (324.5, 120.5) -> (324.5, 117.5)
  line L8 (324.5, 128.5) -> (326.5, 128.5)
  line L9 (326.5, 128.5) -> (326.5, 131.5)
  line L10 (326.5, 131.5) -> (324.5, 131.5)
  line L11 (324.5, 131.5) -> (324.5, 128.5)
  line L12 (324.5, 139.5) -> (326.5, 139.5)
  line L13 (326.5, 139.5) -> (326.5, 142.5)
  line L14 (326.5, 142.5) -> (324.5, 142.5)
  line L15 (324.5, 142.5) -> (324.5, 139.5)
  line L16 (324.5, 150.5) -> (326.5, 150.5)
  line L17 (326.5, 150.5) -> (326.5, 153.5)
  line L18 (326.5, 153.5) -> (324.5, 153.5)
  line L19 (324.5, 153.5) -> (324.5, 150.5)
extrude "side_vent native extrusion (11)" add sketch "side_vent profile (11)" along normal blind 5 separate body makes body 299 at (324.5, 141.5, 27.1667) makes body 300 at (324.5, 130.5, 27.1667) makes body 301 at (324.5, 119.5, 27.1667) makes body 302 at (324.5, 108.5, 27.1667) makes body 303 at (324.5, 152.5, 27.1667) in component "enclosure | Enclosure - revised silhouette | revision 0.3"
ref_plane "WorkPlane22" through (0, 0, 53.5) normal (0, 0, 1) x (1, 0, 0) in component "enclosure | Enclosure - revised silhouette | revision 0.3"
sketch "side_vent profile (12)" plane through (0, 0, 53.5) normal (0, 0, 1) x (1, 0, 0) in component "enclosure | Enclosure - revised silhouette | revision 0.3"
  line L0 (324.5, 106.5) -> (326.5, 106.5)
  line L1 (326.5, 106.5) -> (326.5, 109.5)
  line L2 (326.5, 109.5) -> (324.5, 109.5)
  line L3 (324.5, 109.5) -> (324.5, 106.5)
  line L4 (324.5, 117.5) -> (326.5, 117.5)
  line L5 (326.5, 117.5) -> (326.5, 120.5)
  line L6 (326.5, 120.5) -> (324.5, 120.5)
  line L7 (324.5, 120.5) -> (324.5, 117.5)
  line L8 (324.5, 128.5) -> (326.5, 128.5)
  line L9 (326.5, 128.5) -> (326.5, 131.5)
  line L10 (326.5, 131.5) -> (324.5, 131.5)
  line L11 (324.5, 131.5) -> (324.5, 128.5)
  line L12 (324.5, 139.5) -> (326.5, 139.5)
  line L13 (326.5, 139.5) -> (326.5, 142.5)
  line L14 (326.5, 142.5) -> (324.5, 142.5)
  line L15 (324.5, 142.5) -> (324.5, 139.5)
  line L16 (324.5, 150.5) -> (326.5, 150.5)
  line L17 (326.5, 150.5) -> (326.5, 153.5)
  line L18 (326.5, 153.5) -> (324.5, 153.5)
  line L19 (324.5, 153.5) -> (324.5, 150.5)
extrude "side_vent native extrusion (12)" add sketch "side_vent profile (12)" along normal blind 5 separate body makes body 304 at (324.5, 141.5, 55.1667) makes body 305 at (324.5, 130.5, 55.1667) makes body 306 at (324.5, 119.5, 55.1667) makes body 307 at (324.5, 108.5, 55.1667) makes body 308 at (324.5, 152.5, 55.1667) in component "enclosure | Enclosure - revised silhouette | revision 0.3"
ref_plane "WorkPlane23" through (0, 0, 81.5) normal (0, 0, 1) x (1, 0, 0) in component "enclosure | Enclosure - revised silhouette | revision 0.3"
sketch "side_vent profile (13)" plane through (0, 0, 81.5) normal (0, 0, 1) x (1, 0, 0) in component "enclosure | Enclosure - revised silhouette | revision 0.3"
  line L0 (324.5, 106.5) -> (326.5, 106.5)
  line L1 (326.5, 106.5) -> (326.5, 109.5)
  line L2 (326.5, 109.5) -> (324.5, 109.5)
  line L3 (324.5, 109.5) -> (324.5, 106.5)
  line L4 (324.5, 117.5) -> (326.5, 117.5)
  line L5 (326.5, 117.5) -> (326.5, 120.5)
  line L6 (326.5, 120.5) -> (324.5, 120.5)
  line L7 (324.5, 120.5) -> (324.5, 117.5)
  line L8 (324.5, 128.5) -> (326.5, 128.5)
  line L9 (326.5, 128.5) -> (326.5, 131.5)
  line L10 (326.5, 131.5) -> (324.5, 131.5)
  line L11 (324.5, 131.5) -> (324.5, 128.5)
  line L12 (324.5, 139.5) -> (326.5, 139.5)
  line L13 (326.5, 139.5) -> (326.5, 142.5)
  line L14 (326.5, 142.5) -> (324.5, 142.5)
  line L15 (324.5, 142.5) -> (324.5, 139.5)
  line L16 (324.5, 150.5) -> (326.5, 150.5)
  line L17 (326.5, 150.5) -> (326.5, 153.5)
  line L18 (326.5, 153.5) -> (324.5, 153.5)
  line L19 (324.5, 153.5) -> (324.5, 150.5)
extrude "side_vent native extrusion (13)" add sketch "side_vent profile (13)" along normal blind 5 separate body makes body 309 at (324.5, 141.5, 83.1667) makes body 310 at (324.5, 130.5, 83.1667) makes body 311 at (324.5, 119.5, 83.1667) makes body 312 at (324.5, 108.5, 83.1667) makes body 313 at (324.5, 152.5, 83.1667) in component "enclosure | Enclosure - revised silhouette | revision 0.3"
ref_plane "WorkPlane1" through (0, 0, 347) normal (0, 0, 1) x (1, 0, 0) in component "front_controls | Front control strip | revision 0.3"
sketch "control_recess profile" plane through (0, 0, 347) normal (0, 0, 1) x (1, 0, 0) in component "front_controls | Front control strip | revision 0.3"
  line L0 (-219, 51) -> (-35, 51)
  line L1 (-35, 51) -> (-35, 87)
  line L2 (-35, 87) -> (-219, 87)
  line L3 (-219, 87) -> (-219, 51)
extrude "control_recess native extrusion" add sketch "control_recess profile" along normal blind 4 separate body makes body 314 in component "front_controls | Front control strip | revision 0.3"
ref_plane "WorkPlane2" through (0, 0, 351.5) normal (0, 0, 1) x (1, 0, 0) in component "front_controls | Front control strip | revision 0.3"
sketch "led_0 profile" plane through (0, 0, 351.5) normal (0, 0, 1) x (1, 0, 0) in component "front_controls | Front control strip | revision 0.3"
  line L0 (-141.5, 68.5) -> (-132.5, 68.5)
  line L1 (-132.5, 68.5) -> (-132.5, 77.5)
  line L2 (-132.5, 77.5) -> (-141.5, 77.5)
  line L3 (-141.5, 77.5) -> (-141.5, 68.5)
extrude "led_0 native extrusion" add sketch "led_0 profile" along normal blind 3 separate body makes body 315 in component "front_controls | Front control strip | revision 0.3"
ref_plane "WorkPlane3" through (0, 0, 351.5) normal (0, 0, 1) x (1, 0, 0) in component "front_controls | Front control strip | revision 0.3"
sketch "led_1 profile" plane through (0, 0, 351.5) normal (0, 0, 1) x (1, 0, 0) in component "front_controls | Front control strip | revision 0.3"
  line L0 (-98.5, 68.5) -> (-89.5, 68.5)
  line L1 (-89.5, 68.5) -> (-89.5, 77.5)
  line L2 (-89.5, 77.5) -> (-98.5, 77.5)
  line L3 (-98.5, 77.5) -> (-98.5, 68.5)
extrude "led_1 native extrusion" add sketch "led_1 profile" along normal blind 3 separate body makes body 316 in component "front_controls | Front control strip | revision 0.3"
ref_plane "WorkPlane4" through (0, 0, 351.5) normal (0, 0, 1) x (1, 0, 0) in component "front_controls | Front control strip | revision 0.3"
sketch "led_2 profile" plane through (0, 0, 351.5) normal (0, 0, 1) x (1, 0, 0) in component "front_controls | Front control strip | revision 0.3"
  line L0 (-55.5, 68.5) -> (-46.5, 68.5)
  line L1 (-46.5, 68.5) -> (-46.5, 77.5)
  line L2 (-46.5, 77.5) -> (-55.5, 77.5)
  line L3 (-55.5, 77.5) -> (-55.5, 68.5)
extrude "led_2 native extrusion" add sketch "led_2 profile" along normal blind 3 separate body makes body 317 in component "front_controls | Front control strip | revision 0.3"
ref_plane "WorkPlane5" through (0, 0, 349.5) normal (0, 0, 1) x (1, 0, 0) in component "front_controls | Front control strip | revision 0.3"
sketch "power_switch profile" plane through (0, 0, 349.5) normal (0, 0, 1) x (1, 0, 0) in component "front_controls | Front control strip | revision 0.3"
  line L0 (-204, 62) -> (-184, 62)
  line L1 (-184, 62) -> (-184, 84)
  line L2 (-184, 84) -> (-204, 84)
  line L3 (-204, 84) -> (-204, 62)
extrude "power_switch native extrusion" add sketch "power_switch profile" along normal blind 7 separate body makes body 318 in component "front_controls | Front control strip | revision 0.3"
ref_plane "WorkPlane1" through (0, 0, -325) normal (0, 0, 1) x (1, 0, 0) in component "rear_interfaces | Rear connections | revision 0.3"
sketch "connector_0 profile" plane through (0, 0, -325) normal (0, 0, 1) x (1, 0, 0) in component "rear_interfaces | Rear connections | revision 0.3"
  line L0 (-154, 161.5) -> (-126, 161.5)
  line L1 (-126, 161.5) -> (-126, 178.5)
  line L2 (-126, 178.5) -> (-154, 178.5)
  line L3 (-154, 178.5) -> (-154, 161.5)
extrude "connector_0 native extrusion" add sketch "connector_0 profile" along normal blind 6 separate body makes body 319 in component "rear_interfaces | Rear connections | revision 0.3"
ref_plane "WorkPlane2" through (0, 0, -325) normal (0, 0, 1) x (1, 0, 0) in component "rear_interfaces | Rear connections | revision 0.3"
sketch "connector_1 profile" plane through (0, 0, -325) normal (0, 0, 1) x (1, 0, 0) in component "rear_interfaces | Rear connections | revision 0.3"
  line L0 (-94, 161.5) -> (-66, 161.5)
  line L1 (-66, 161.5) -> (-66, 178.5)
  line L2 (-66, 178.5) -> (-94, 178.5)
  line L3 (-94, 178.5) -> (-94, 161.5)
extrude "connector_1 native extrusion" add sketch "connector_1 profile" along normal blind 6 separate body makes body 320 in component "rear_interfaces | Rear connections | revision 0.3"
ref_plane "WorkPlane3" through (0, 0, -325) normal (0, 0, 1) x (1, 0, 0) in component "rear_interfaces | Rear connections | revision 0.3"